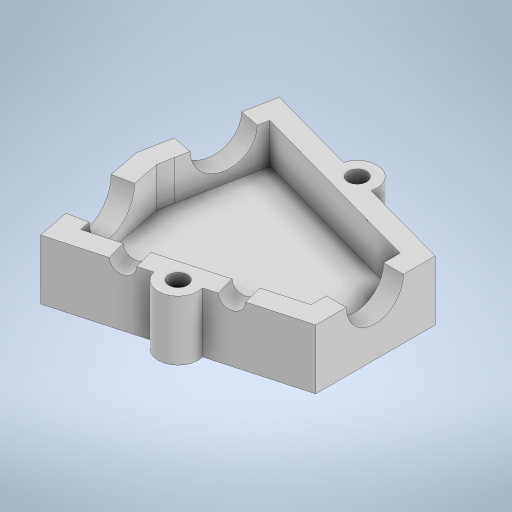
# Autodesk Inventor part: powerFromBatterySplitHousing
Saved by Autodesk Inventor 2024 (Build 280153000, 153)
## iProperties
Created: 2023-08-08
Part Number: powerFromBatterySplitHousing
Material: Generic
Document SubType Name: Modeling
Designer: 18179
Density: 1 g/cm^3
Appearance: Default
Author: 18179
Autodesk Inventor part; units mm, degrees
ref_plane "YZ Plane" through (0, 0, 0) normal (1, 0, 0) x (0, 1, 0)
ref_plane "XZ Plane" through (0, 0, 0) normal (0, 1, 0) x (-1, 0, 0)
ref_plane "XY Plane" through (0, 0, 0) normal (0, 0, 1) x (1, 0, 0)
sketch "Sketch1" plane through (0, 0, 0) normal (0, 1, 0) x (-1, 0, 0)
  line L0 (0, 0) -> (25.4, 0)
  line L1 (25.4, 0) -> (25.4, -19.05)
  line L2 (25.4, -19.05) -> (0, -19.05)
  line L3 (0, -19.05) -> (0, 0)
  line L4 (25.4, -9.525) -> (38.1, -9.525)
  line L5 (38.1, -9.525) -> (34.3696, 9.525)
  line L6 (34.3696, 9.525) -> (0, 0)
  line L7 (38.1, -9.525) -> (34.3696, -28.575)
  line L8 (34.3696, -28.575) -> (0, -19.05)
  line L9 (-0.8514, -15.5194) -> (31.9128, -24.5995)
  line L10 (31.9128, -24.5995) -> (34.3908, -11.9449)
  line L11 (1.5358, -2.8691) -> (31.9128, 5.5495)
  line L12 (31.9128, 5.5495) -> (34.3903, -7.1024)
  line L13 (3.175, -19.05) -> (3.175, -6.35)
  line L14 (34.3908, -11.9449) -> (38.1, 8.3994)
  line L15 (34.3903, -7.1024) -> (39.9584, -35.5367)
  line L16 (3.175, -6.35) -> (3.175, -2.4148)
  point P0 (3.175, -19.05)
  point P1 (3.175, 0)
  point P2 (11.8883, 0)
  point P3 (34.7909, -6.35)
  point P4 (11.8883, -19.05)
  point P5 (3.175, -16.6352)
  point P6 (3.175, -2.6421)
  point P7 (0, -15.7553)
  point P8 (34.8478, -9.4386)
  dimension "d0" = 25.4
  dimension "d1" = 19.05
  dimension "d2" = 12.7
  dimension "d3" = 19.05
  dimension "d4" = 3.175
  dimension "d5" = 3.175
  dimension "d6" = 3.175
  constraints: 34 end point, 4 parallel, 2 horizontal, 1 midpoint, 1 perpendicular, 1 point on line, 1 symmetric about line, 1 vertical, 2 other
  measures "d0" distance of L1.end L2.end
  measures "d1" distance of L0.end L1.end
  measures "d2" distance of L4.start L4.end
  measures "d3" vertical distance of L5.end L4.end
  measures "d4" distance between parallel lines of L8 L9
  measures "d5" distance between parallel lines of L6 L11
  measures "d6" distance between parallel lines of L3 L13
extrude "Extrusion1" add sketch "Sketch1" against normal blind 9.525 contours L6 L5 L14 L15 L12 L11 L0 | L0 L11 L16 L13 L9 L3 | L9 L13 L2 L3 | L2 L9 L10 L14 L4 L15 L7 L8 | L9 L2 L13 | L5 L4 L15 L14 | L7 L15 L4 | L15 L4 L14
sketch "Sketch3" plane through (-38.1, -9.525, -9.525) normal (-0.9814, 0, 0.1922) x (0.1922, 0, 0.9814)
  line L0 (0, 9.525) -> (19.4118, 9.525) projected
  circle A0 centre (9.7059, 9.525) radius 4.572
  point P0 (16.6692, 9.525)
  point P1 (14.2779, 9.525)
  point P2 (5.1339, 9.525)
  dimension "d12" = 9.144
  constraints: 1 centre point, 1 midpoint
  measures "d12" diameter of A0
extrude "Extrusion3" cut sketch "Sketch3" against normal blind 25.4 contours L0 A0 picked at (10.7462, 7.5625)
sketch "Sketch4" plane through (-34.3696, -9.525, -28.575) normal (-0.9814, 0, -0.1922) x (-0.1922, 0, 0.9814)
  line L0 (0, 9.525) -> (19.4118, 9.525) projected
  circle A0 centre (9.7059, 9.525) radius 4.572
  point P0 (21.4375, 9.525)
  point P1 (14.2779, 9.525)
  point P2 (5.1339, 9.525)
  dimension "d15" = 9.144
  constraints: 1 centre point, 1 midpoint
  measures "d15" diameter of A0
extrude "Extrusion4" cut sketch "Sketch4" against normal blind 25.4 contours L0 A0 picked at (10.7462, 7.5625)
sketch "Sketch5" plane through (-3.175, 0, -16.6352) normal (-1, 0, 0) x (0, 0, 1)
  line L0 (7.1966, 0) -> (4.6903, 0) projected
  circle A0 centre (7.1966, 0) radius 4.572
  point P0 (16.6352, 0)
  dimension "d18" = 9.144
  constraints: 1 centre point
  measures "d18" diameter of A0
extrude "Extrusion5" cut sketch "Sketch5" against normal blind 9.525
sketch "Sketch6" plane through (0, -9.525, 0) normal (0, -1, 0) x (1, 0, 0)
  line L0 (-34.3696, -28.575) -> (0, -19.05) projected
  line L1 (0, -19.05) -> (0, 0) projected
  line L2 (0, 0) -> (-34.3696, 9.525) projected
  line L3 (-34.3696, 9.525) -> (-38.1, -9.525) projected
  line L4 (-38.1, -9.525) -> (-34.3696, -28.575) projected
  line L5 (-3.175, -2.4148) -> (-3.175, -16.6352) projected
  line L6 (-3.175, -16.6352) -> (-31.9128, -24.5995) projected
  line L7 (-31.9128, -24.5995) -> (-34.3908, -11.9449) projected
  line L8 (-34.3908, -11.9449) -> (-34.8478, -9.4386) projected
  line L9 (-34.8478, -9.4386) -> (-31.9128, 5.5495) projected
  line L10 (-31.9128, 5.5495) -> (-3.175, -2.4148) projected
extrude "Extrusion6" add sketch "Sketch6" against normal blind 3.175 contours L4 L3 L2 L1 L0 | L5 L6 L7 L8 L9 L10
sketch "Sketch7" plane through (0, 0, 0) normal (0, 1, 0) x (1, 0, 0)
  line L0 (-34.3696, -9.525) -> (0, 0) projected
  circle A0 centre (-17.1848, -4.7625) radius 3.175
  line L1 (-10.5511, 0.3706) -> (-31.9128, -5.5495) projected
  line L2 (-34.3696, 28.575) -> (0, 19.05) projected
  circle A1 centre (-17.1848, 23.8125) radius 3.175
  line L3 (-31.9128, 24.5995) -> (-10.5511, 18.6794) projected
  point P0 (-20.2445, 24.6604)
  point P1 (-14.1251, 22.9646)
  point P2 (-14.1251, -3.9146)
  point P3 (-20.2445, -5.6104)
  constraints: 2 centre point, 2 midpoint, 2 tangent
extrude "Extrusion7" add sketch "Sketch7" against normal blind 9.525 contours L0 A0 | A1 L2 picked at (-16.7975, -6.2491) picked at (-16.3793, 25.0421)
sketch "Sketch8" plane through (0, 0, 0) normal (0, 1, 0) x (1, 0, 0)
  arc A0 (-14.1251, 22.9646) -> (-20.2445, 24.6604) centre (-17.1848, 23.8125) ccw projected
  circle A1 centre (-17.1848, 23.8125) radius 1.5
  arc A2 (-20.2445, -5.6104) -> (-14.1251, -3.9146) centre (-17.1848, -4.7625) ccw projected
  circle A3 centre (-17.1848, -4.7625) radius 1.5
  point P0 (0, 0)
  dimension "d25" = 3
  dimension "d26" = 3
  constraints: 2 centre point, 2 coincident
  measures "d25" diameter of A1
  measures "d26" diameter of A3
extrude "Extrusion8" cut sketch "Sketch8" against normal blind 9.525
sketch "Sketch10" plane through (-34.3696, -9.525, 9.525) normal (0.2671, 0, 0.9637) x (0.9637, 0, -0.2671)
  line L0 (25.5962, 9.525) -> (3.4293, 9.525) projected
  circle A0 centre (10.7027, 9.525) radius 1.778
  circle A1 centre (24.8175, 9.525) radius 1.778
  line L1 (21.0075, 9.525) -> (21.0075, 0) projected
  point P0 (35.665, 9.525)
  point P1 (14.5127, 9.525)
  point P2 (8.9247, 9.525)
  point P3 (12.4807, 9.525)
  dimension "d29" = 3.556
  dimension "d30" = 3.556
  dimension "d31" = 3.81
  dimension "d32" = 3.81
  constraints: 2 centre point, 2 point on line, 1 midpoint
  measures "d29" diameter of A0
  measures "d30" diameter of A1
  measures "d31" distance of point (14.513, 9.525) A0.centre
  measures "d32" distance from line of L1 A1.centre
extrude "Extrusion9" cut sketch "Sketch10" against normal blind 9.525 contours A0 L0 | A1 picked at (11.0394, 9.0372)
body "Solid1"
